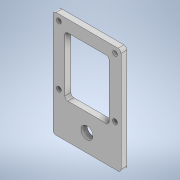
# Autodesk Inventor part: 2 Stage Climber in a box bracket
Saved by Autodesk Inventor 2022 (Build 260153000, 153)
## iProperties
Created: 2022-02-13
Part Number: 2 Stage Climber in a box bracket
Material: Generic
Document SubType Name: Modeling
Designer: hawle
Density: 1 g/cm^3
Appearance: Default
Author: hawle
Autodesk Inventor part; units mm, degrees
ref_plane "YZ Plane" through (0, 0, 0) normal (1, 0, 0) x (0, 1, 0)
ref_plane "XZ Plane" through (0, 0, 0) normal (0, 1, 0) x (-1, 0, 0)
ref_plane "XY Plane" through (0, 0, 0) normal (0, 0, 1) x (1, 0, 0)
sketch "Sketch1" plane through (0, 0, 0) normal (0, 0, 1) x (1, 0, 0)
  line L0 (17.6686, 31.4113) -> (84.3436, 31.4113)
  line L1 (87.5186, 28.2363) -> (87.5186, -44.7887)
  line L2 (14.4936, -44.7887) -> (14.4936, 28.2363)
  line L3 (30.3686, 18.7113) -> (71.6436, 18.7113)
  line L4 (74.8186, 15.5363) -> (74.8186, -41.6137)
  line L5 (27.1936, 15.5363) -> (27.1936, -41.6137)
  circle A0 centre (20.8436, 25.0613) radius 2.5527
  circle A1 centre (81.1686, 25.0613) radius 2.5527
  arc A2 (17.6686, 31.4113) -> (14.4936, 28.2363) centre (17.6686, 28.2363) ccw
  arc A3 (87.5186, 28.2363) -> (84.3436, 31.4113) centre (84.3436, 28.2363) ccw
  circle A4 centre (20.8436, -38.4387) radius 2.5527
  circle A5 centre (81.1686, -38.4387) radius 2.5527
  line L6 (30.3686, -44.7887) -> (71.6436, -44.7887)
  line L7 (87.5186, -44.7887) -> (87.5186, -79.7137)
  line L8 (84.3436, -82.8887) -> (17.6686, -82.8887)
  line L9 (14.4936, -79.7137) -> (14.4936, -44.7887)
  circle A6 centre (51.0061, -63.8387) radius 6.35
  arc A7 (14.4936, -79.7137) -> (17.6686, -82.8887) centre (17.6686, -79.7137) ccw
  arc A8 (84.3436, -82.8887) -> (87.5186, -79.7137) centre (84.3436, -79.7137) ccw
  arc A9 (71.6436, -44.7887) -> (74.8186, -41.6137) centre (71.6436, -41.6137) ccw
  arc A10 (27.1936, -41.6137) -> (30.3686, -44.7887) centre (30.3686, -41.6137) ccw
  arc A11 (30.3686, 18.7113) -> (27.1936, 15.5363) centre (30.3686, 15.5363) ccw
  arc A12 (74.8186, 15.5363) -> (71.6436, 18.7113) centre (71.6436, 15.5363) ccw
  point P0 (0, 0)
  point P1 (87.5186, 31.4113)
  dimension "d1" = 76.2
  dimension "d2" = 73.025
  dimension "d3" = 12.7
  dimension "d4" = 12.7
  dimension "d5" = 12.7
  dimension "d6" = 5.1054
  dimension "d7" = 6.35
  dimension "d9" = 5.1054
  dimension "d10" = 6.35
  dimension "d11" = 6.35
  dimension "d12" = 3.175
  dimension "d13" = 5.1054
  dimension "d14" = 5.1054
  dimension "d15" = 63.5
  dimension "d16" = 63.5
  dimension "d17" = 76.2
  dimension "d18" = 12.7
  dimension "d19" = 36.5125
  dimension "d20" = 38.1
  dimension "d21" = 19.05
  dimension "d22" = 3.175
  dimension "d23" = 3.175
  dimension "d26" = 60.325
  dimension "d27" = 0
  constraints: 20 end point, 16 point on circle, 16 tangent, 13 centre point, 5 equal radius, 4 point on line, 3 horizontal, 3 parallel, 3 perpendicular, 1 vertical
  measures "d1" distance of point (87.519, 31.411) L1.end
  measures "d2" distance between parallel lines of L2 L1
  measures "d3" distance between parallel lines of L3 L0
  measures "d4" distance between parallel lines of L5 L2
  measures "d5" distance between parallel lines of L1 L4
  measures "d6" diameter of A0
  measures "d7" distance from line of L0 A0.centre
  measures "d9" diameter of A1
  measures "d10" distance from line of A1.centre L0
  measures "d11" distance from line of L1 A1.centre
  measures "d12" radius of A2
  measures "d13" diameter of A4
  measures "d14" diameter of A5
  measures "d15" distance of A4.centre A0.centre
  measures "d16" distance of A5.centre A1.centre
  measures "d17" distance between parallel lines of L6 L0
  measures "d18" diameter of A6
  measures "d19" distance from line of L9 A6.centre
  measures "d20" distance between parallel lines of L8 L6
  measures "d21" distance from line of L8 A6.centre
  measures "d22" radius of A7
  measures "d23" radius of A11
  measures "d26" distance of A0.centre A1.centre
  measures "d27" distance between parallel lines of L1 L7
extrude "Extrusion1" add sketch "Sketch1" along normal blind 6.35
body "Solid1"
